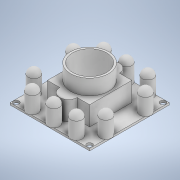
# Autodesk Inventor part: new camera'
Saved by Autodesk Inventor 2020 (Build 240168000, 168)
## iProperties
Created: 2019-07-23
Part Number: new camera'
Material: Generic
Document SubType Name: Modeling
Designer: Paul
Density: 1 g/cm^3
Appearance: Default
Author: Paul
Autodesk Inventor part; units mm, degrees
ref_plane "YZ Plane" through (0, 0, 0) normal (1, 0, 0) x (0, 1, 0)
ref_plane "XZ Plane" through (0, 0, 0) normal (0, 1, 0) x (-1, 0, 0)
ref_plane "XY Plane" through (0, 0, 0) normal (0, 0, 1) x (1, 0, 0)
sketch "Sketch1" plane through (0, 0, 0) normal (0, 1, 0) x (-1, 0, 0)
  line L0 (16, 16) -> (-16, 16)
  line L1 (-16, 16) -> (-16, -16)
  line L2 (-16, -16) -> (16, -16)
  line L3 (16, -16) -> (16, 16)
  line L4 (16, 16) -> (-16, -16) construction
  line L5 (-16, 16) -> (16, -16) construction
  point P0 (0, 0)
  dimension "d0" = 32
  dimension "d1" = 32
  constraints: 12 end point, 2 midpoint, 2 parallel, 1 horizontal, 1 perpendicular
  measures "d0" distance of L2.end L1.end
  measures "d1" distance of L1.end L0.end
extrude "Extrusion1" add sketch "Sketch1" along normal blind 0.85
sketch "Sketch2" plane through (0, 0.85, 0) normal (0, 1, 0) x (1, 0, 0)
  line L0 (-8.5, 8.5) -> (8.5, 8.5)
  line L1 (8.5, 8.5) -> (8.5, -8.5)
  line L2 (8.5, -8.5) -> (-8.5, -8.5)
  line L3 (-8.5, -8.5) -> (-8.5, 8.5)
  line L4 (-8.5, 8.5) -> (8.5, -8.5) construction
  line L5 (8.5, 8.5) -> (-8.5, -8.5) construction
  circle A0 centre (0, 8.5) radius 3.5
  circle A1 centre (0, -8.5) radius 3.5
  point P0 (0, 0)
  point P1 (3.5, 8.5)
  point P2 (-3.5, 8.5)
  point P3 (-3.5, -8.5)
  point P4 (3.5, -8.5)
  dimension "d4" = 17
  dimension "d5" = 17
  dimension "d6" = 7
  dimension "d7" = 7
  constraints: 12 end point, 4 midpoint, 2 centre point, 2 parallel, 1 horizontal, 1 perpendicular
  measures "d4" distance of L1.end L2.end
  measures "d5" distance of L0.end L1.end
  measures "d6" diameter of A0
  measures "d7" diameter of A1
extrude "Extrusion2" add sketch "Sketch2" along normal blind 7.75
sketch "Sketch3" plane through (0, 8.6, 0) normal (0, 1, 0) x (1, 0, 0)
  circle A0 centre (0, 0) radius 7.66
  dimension "d10" = 15.32
  constraints: 1 centre point, 1 coincident
  measures "d10" diameter of A0
extrude "Extrusion3" add sketch "Sketch3" along normal blind 6.17
sketch "Sketch4" plane through (0, 14.77, 0) normal (0, 1, 0) x (1, 0, 0)
  circle A0 centre (0, 0) radius 6.85
  dimension "d13" = 13.7
  constraints: 1 centre point, 1 coincident
  measures "d13" diameter of A0
extrude "Extrusion4" cut sketch "Sketch4" against normal blind 13.92
sketch "Sketch5" plane through (0, 0.85, 0) normal (0, 1, 0) x (1, 0, 0)
  point P0 (0, 0)
sketch "Sketch6" plane through (0, 0, 0) normal (0, -1, 0) x (1, 0, 0)
  line L0 (16, 16) -> (16, -16) projected
  line L1 (-16, 16) -> (16, 16) projected
  circle A0 centre (-14.76, 14.76) radius 1.11
  circle A1 centre (14.76, -14.76) radius 1.11
  line L2 (16, -16) -> (-16, -16) projected
  circle A2 centre (14.76, 14.76) radius 1.11
  circle A3 centre (-14.76, -14.76) radius 1.11
  point P0 (0, 0)
  dimension "d23" = 2.22
  dimension "d24" = 2.22
  dimension "d26" = 1.24
  dimension "d28" = 1.24
  dimension "d29" = 1.24
  dimension "d30" = 2.22
  dimension "d31" = 2.22
  constraints: 4 centre point
  measures "d23" diameter of A0
  measures "d24" diameter of A1
  measures "d26" distance from line of L1 A0.centre
  measures "d28" distance from line of L2 A1.centre
  measures "d29" distance from line of L0 A1.centre
  measures "d30" diameter of A2
  measures "d31" diameter of A3
extrude "Extrusion5" cut sketch "Sketch6" against normal blind 0.85
sketch "Sketch9" plane through (0, 0.85, 0) normal (0, 1, 0) x (1, 0, 0)
  circle A0 centre (-8.9, 14.5) radius 2.3
  line L0 (16, 16) -> (-16, 16) projected
  line L1 (-16, 16) -> (-16, -16) projected
  circle A1 centre (8.9, 14.5) radius 2.3
  line L2 (16, -16) -> (16, 16) projected
  point P0 (0, 0)
  dimension "d34" = 4.6
  dimension "d35" = 1.5
  dimension "d36" = 7.1
  dimension "d37" = 4.6
  dimension "d38" = 1.5
  dimension "d39" = 7.1
  constraints: 2 centre point
  measures "d34" diameter of A0
  measures "d35" distance from line of L0 A0.centre
  measures "d36" distance from line of L1 A0.centre
  measures "d37" diameter of A1
  measures "d38" distance from line of L0 A1.centre
  measures "d39" distance from line of L2 A1.centre
sketch "Sketch10" plane through (0, 0.85, 0) normal (0, 1, 0) x (1, 0, 0)
  circle A0 centre (0, 14.7) radius 2.3
  line L0 (16, 16) -> (-16, 16) projected
  line L1 (16, -16) -> (16, 16) projected
  point P0 (0, 0)
  dimension "d40" = 4.6
  dimension "d41" = 1.3
  dimension "d42" = 16
  constraints: 1 centre point
  measures "d40" diameter of A0
  measures "d41" distance from line of L0 A0.centre
  measures "d42" distance from line of L1 A0.centre
sketch "Sketch11" plane through (0, 0.85, 0) normal (0, 1, 0) x (1, 0, 0)
  circle A0 centre (-8.9, -14.2) radius 2.3
  circle A1 centre (0, -14.4) radius 2.3
  circle A2 centre (8.9, -14.2) radius 2.3
  circle A3 centre (-14.5, 7.96) radius 2.3
  circle A4 centre (14.5, 7.96) radius 2.3
  circle A5 centre (14.5, -7.96) radius 2.3
  circle A6 centre (-14.5, -7.96) radius 2.3
  line L0 (16, 16) -> (-16, 16) projected
  line L1 (16, -16) -> (16, 16) projected
  line L2 (-16, -16) -> (16, -16) projected
  line L3 (-16, 16) -> (-16, -16) projected
  point P0 (0, 0)
  dimension "d43" = 4.6
  dimension "d44" = 4.6
  dimension "d45" = 4.6
  dimension "d46" = 4.6
  dimension "d47" = 4.6
  dimension "d48" = 4.6
  dimension "d49" = 4.6
  dimension "d50" = 8.04
  dimension "d51" = 1.5
  dimension "d52" = 8.04
  dimension "d53" = 1.5
  dimension "d54" = 8.04
  dimension "d55" = 1.5
  dimension "d56" = 1.5
  dimension "d57" = 8.04
  dimension "d58" = 7.1
  dimension "d59" = 1.8
  dimension "d60" = 7.1
  dimension "d61" = 1.8
  dimension "d62" = 16
  dimension "d63" = 1.6
  constraints: 7 centre point
  measures "d43" diameter of A0
  measures "d44" diameter of A1
  measures "d45" diameter of A2
  measures "d46" diameter of A3
  measures "d47" diameter of A4
  measures "d48" diameter of A5
  measures "d49" diameter of A6
  measures "d50" distance from line of L0 A4.centre
  measures "d51" distance from line of L1 A4.centre
  measures "d52" distance from line of L2 A5.centre
  measures "d53" distance from line of L1 A5.centre
  measures "d54" distance from line of L0 A3.centre
  measures "d55" distance from line of L3 A3.centre
  measures "d56" distance from line of L3 A6.centre
  measures "d57" distance from line of L2 A6.centre
  measures "d58" distance from line of L3 A0.centre
  measures "d59" distance from line of L2 A0.centre
  measures "d60" distance from line of L1 A2.centre
  measures "d61" distance from line of L2 A2.centre
  measures "d62" distance from line of L1 A1.centre
  measures "d63" distance from line of L2 A1.centre
extrude "Extrusion6" add sketch "Sketch11" along normal blind 9 contours A0 L2 | L2 A0 | L2 A1 | A1 L2 | L3 A6 | A6 L3 | L2 A2 | A2 L2 | L3 A3 | A3 L3 | L1 A5 | A5 L1 | L1 A4 | A4 L1
extrude "Extrusion7" add sketch "Sketch9" along normal blind 9
extrude "Extrusion8" add sketch "Sketch10" along normal blind 9
fillet "Fillet1" radius 2.3 10 edges at (6.6, 9.85, -14.5) (-2.3, 9.85, -14.7) (-11.2, 9.85, -14.5) (-16.8, 9.85, -7.96) (-16.8, 9.85, 7.96) (-11.2, 9.85, 14.2) (-2.3, 9.85, 14.4) (6.6, 9.85, 14.2) (12.2, 9.85, 7.96) (12.2, 9.85, -7.96)
sketch "Sketch12" plane through (0, 0, 0) normal (0, -1, 0) x (1, 0, 0)
  line L0 (-16, -3.7) -> (-12.3, -3.7)
  line L1 (-12.3, -3.7) -> (-12.3, 3.7)
  line L2 (-12.3, 3.7) -> (-16, 3.7)
  line L3 (-16, 3.7) -> (-16, -3.7)
  line L4 (-16, -3.7) -> (-12.3, 3.7) construction
  line L5 (-12.3, -3.7) -> (-16, 3.7) construction
  line L6 (-16, -16) -> (-16, 16) projected
  line L7 (-16, 16) -> (16, 16) projected
  point P0 (0, 0)
  point P1 (-14.15, 0)
  dimension "d71" = 3.7
  dimension "d72" = 7.4
  dimension "d73" = 0
  dimension "d74" = 12.3
  constraints: 12 end point, 2 midpoint, 2 parallel, 1 horizontal, 1 perpendicular
  measures "d71" distance of L2.end L1.end
  measures "d72" distance of L1.end L0.end
  measures "d73" distance between parallel lines of L6 L3
  measures "d74" distance between parallel lines of L7 L2
extrude "Extrusion9" add sketch "Sketch12" along normal blind 4.45
sketch "Sketch13" plane through (0, -4.45, 0) normal (0, -1, 0) x (1, 0, 0)
  line L0 (-15.7, 3.4) -> (-12.6, 3.4)
  line L1 (-12.6, 3.4) -> (-12.6, -3.4)
  line L2 (-12.6, -3.4) -> (-15.7, -3.4)
  line L3 (-15.7, -3.4) -> (-15.7, 3.4)
  line L4 (-15.7, 3.4) -> (-12.6, -3.4) construction
  line L5 (-12.6, 3.4) -> (-15.7, -3.4) construction
  line L6 (-16, 3.7) -> (-16, -3.7) projected
  line L7 (-12.3, 3.7) -> (-16, 3.7) projected
  point P0 (0, 0)
  point P1 (-14.15, 0)
  dimension "d77" = 3.1
  dimension "d78" = 6.8
  dimension "d79" = 0.3
  dimension "d80" = 0.3
  constraints: 12 end point, 2 midpoint, 2 parallel, 1 horizontal, 1 perpendicular
  measures "d77" distance of L1.end L2.end
  measures "d78" distance of L0.end L1.end
  measures "d79" distance between parallel lines of L6 L3
  measures "d80" distance between parallel lines of L7 L0
extrude "Extrusion10" cut sketch "Sketch13" against normal blind 4.4
body "Solid1"
